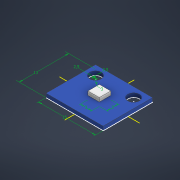
# Autodesk Inventor part: Drucksensor
Saved by Autodesk Inventor 2021 (Build 250183000, 183)
## iProperties
Created: 2020-12-16
Part Number: Drucksensor
Material: Generisch
Document SubType Name: Modeling
Designer: laure
Density: 1 g/cm^3
Appearance: Vorgabe
Author: laure
Autodesk Inventor part; units mm, degrees
ref_plane "YZ Plane" through (0, 0, 0) normal (1, 0, 0) x (0, 1, 0)
ref_plane "XZ Plane" through (0, 0, 0) normal (0, 1, 0) x (-1, 0, 0)
ref_plane "XY Plane" through (0, 0, 0) normal (0, 0, 1) x (1, 0, 0)
sketch "Skizze1" plane through (0, 0, 0) normal (0, 1, 0) x (-1, 0, 0)
  line L0 (7.5, -6.5) -> (-7.5, -6.5)
  line L1 (-7.5, -6.5) -> (-7.5, 6.5)
  line L2 (-7.5, 6.5) -> (7.5, 6.5)
  line L3 (7.5, 6.5) -> (7.5, -6.5)
  line L4 (10.5, 0) -> (-10.5, 0) projected
  line L5 (0, -9.1) -> (0, 9.1) projected
  line L6 (1.5, -1.5) -> (-1.5, -1.5)
  line L7 (-1.5, -1.5) -> (-1.5, 1.5)
  line L8 (-1.5, 1.5) -> (1.5, 1.5)
  line L9 (1.5, 1.5) -> (1.5, -1.5)
  circle A0 centre (5, -4) radius 1.5
  circle A1 centre (-5, -4) radius 1.5
  dimension "d0" = 15
  dimension "d1" = 13
  dimension "d10" = 3
  dimension "d11" = 3
  dimension "d12" = 3
  dimension "d13" = 2.5
  dimension "d14" = 2.5
  constraints: 16 end point, 4 parallel, 2 centre point, 2 horizontal, 2 perpendicular, 1 symmetric about line, 5 other
  measures "d0" distance between parallel lines of L1 L3
  measures "d1" distance between parallel lines of L2 L0
  measures "d10" distance of L7.end L8.end
  measures "d11" distance of L6.end L7.end
  measures "d12" diameter of A0
  measures "d13" distance from line of L0 A0.centre
  measures "d14" distance from line of L3 A0.centre
extrude "Extrusion3" add sketch "Skizze1" along normal blind 1
extrude "Extrusion4" add sketch "Skizze1" along normal blind 2 contours L6 L7 L4 L5 | L5 L4 L9 L6 | L4 L5 L8 L9 | L4 L7 L8 L5
